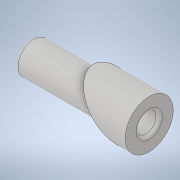
# Autodesk Inventor part: ElectricFenceWasher
Saved by Autodesk Inventor 2020 (Build 240168000, 168)
## iProperties
Created: 2019-06-17
Part Number: ElectricFenceWasher
Material: Generic
Document SubType Name: Modeling
Designer: steele
Density: 1 g/cm^3
Appearance: Default
Author: steele
Autodesk Inventor part; units mm, degrees
ref_plane "XZ Plane" through (0, 0, 0) normal (0, 1, 0) x (-1, 0, 0)
ref_plane "XY Plane" through (0, 0, 0) normal (0, 0, 1) x (1, 0, 0)
ref_plane "Work Plane1" through (0, 0, 0) normal (0.7071068, 0.7071068, 0) x (0, 0, 1)
sketch "Sketch1" plane through (0, 0, 0) normal (1, 0, 0) x (0, 1, 0)
  circle A0 centre (0, 0) radius 19.05
  dimension "outerDiameter" = 38.1
  constraints: 1 centre point, 1 coincident
  measures "outerDiameter" diameter of A0
ref_plane "Work Plane2" through (-12.5724, -12.5724, 0) normal (0.7071068, 0.7071068, 0) x (0, 0, 1)
extrude "Extrusion2" add sketch "Sketch1" against normal up to surface surface through (-12.5724, -12.5724, 0) normal (0.7071068, 0.7071068, 0)
sketch "Sketch3" plane through (0, 0, 0) normal (1, 0, 0) x (0, 0, -1)
  circle A0 centre (0, 0) radius 12.7
  dimension "thruHoleDiameter" = 25.4
  constraints: 1 centre point, 1 coincident
  measures "thruHoleDiameter" diameter of A0
extrude "Extrusion4" add sketch "Sketch3" against normal blind 93.853
sketch "Sketch4" plane through (-93.853, 0, 0) normal (-1, 0, 0) x (0, 0, 1)
  circle A0 centre (0, 0) radius 7.9375
  dimension "holeForString" = 15.875
  constraints: 1 centre point, 1 coincident
  measures "holeForString" diameter of A0
extrude "Extrusion5" cut sketch "Sketch4" against normal through all
fillet "Fillet1" radius 2.54 3 edges at (0, 0, -7.9375) (-93.853, 0, -7.9375) (-93.853, 0, 12.7)
body "Solid2"
